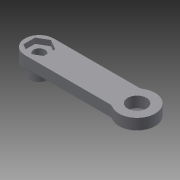
# Autodesk Inventor part: link_long
Saved by Autodesk Inventor 2014 (Build 180170000, 170)
## iProperties
Created: 2015-03-09
Part Number: link_long
Material: 一般
Document SubType Name: Modeling
Designer: Hideyuki Takei
Density: 1 g/cm^3
Appearance: 既定
Author: Hideyuki Takei
Autodesk Inventor part; units mm, degrees
note: some values were not read from the file. Chosen so that the rebuilt part matches the saved one: sketch regions of "押し出し1".
ref_plane "YZ Plane" through (0, 0, 0) normal (1, 0, 0) x (0, 1, 0)
ref_plane "XZ Plane" through (0, 0, 0) normal (0, 1, 0) x (-1, 0, 0)
ref_plane "XY Plane" through (0, 0, 0) normal (0, 0, 1) x (1, 0, 0)
sketch "スケッチ1" plane through (0, 0, 0) normal (0, 0, 1) x (1, 0, 0)
  line L0 (0, 0) -> (27.1, 0) construction
  line L1 (0, -4) -> (27.1, -4)
  line L2 (27.1, 4) -> (0, 4)
  arc A0 (0, 4) -> (0, -4) centre (0, 0) ccw
  arc A1 (27.1, -4) -> (27.1, 4) centre (27.1, 0) ccw
  circle A2 centre (0, 0) radius 1.6
  circle A3 centre (27.1, 0) radius 2.6
  circle A4 centre (27.1, 0) radius 5
  point P0 (13.55, 0)
  dimension "d0" = 27.1
  dimension "d1" = 4
  dimension "d2" = 3.2
  dimension "d3" = 5.2
  dimension "d6" = 10
  constraints: 8 end point, 5 centre point, 4 point on circle, 4 tangent, 3 coincident, 1 horizontal, 1 midpoint, 1 parallel
  measures "d0" distance of L0.start L0.end
  measures "d1" radius of A0
  measures "d2" diameter of A2
  measures "d3" diameter of A3
  measures "d6" diameter of A4
extrude "押し出し1" add sketch "スケッチ1" along normal blind 3
sketch "スケッチ3" plane through (0, 0, 0) normal (0, 0, 1) x (1, 0, 0)
  circle A0 centre (0, 0) radius 4
  circle A1 centre (0, 0) radius 1.6
  dimension "d7" = 8
  dimension "d10" = 3.2
  constraints: 2 centre point, 2 coincident
  measures "d7" diameter of A0
  measures "d10" diameter of A1
extrude "押し出し2" add sketch "スケッチ3" against normal blind 0.5
sketch "スケッチ4" plane through (0, 0, 0) normal (0, 0, 1) x (1, 0, 0)
  circle A0 centre (0, 0) radius 1.6
  circle A1 centre (0, 0) radius 2.5
  dimension "d11" = 5
  dimension "d12" = 3.2
  constraints: 2 centre point, 2 coincident
  measures "d11" diameter of A1
  measures "d12" diameter of A0
extrude "押し出し3" add sketch "スケッチ4" against normal blind 3.7
sketch "スケッチ5" plane through (0, 0, 3) normal (0, 0, 1) x (1, 0, 0)
  circle A0 centre (0, 0) radius 1.6 projected
  arc A1 (0, 4) -> (0, -4) centre (0, 0) ccw projected
  line L0 (0, 3.2332) -> (2.8, 1.6166)
  line L1 (2.8, 1.6166) -> (2.8, -1.6166)
  line L2 (2.8, -1.6166) -> (0, -3.2332)
  line L3 (0, -3.2332) -> (-2.8, -1.6166)
  line L4 (-2.8, -1.6166) -> (-2.8, 1.6166)
  line L5 (-2.8, 1.6166) -> (0, 3.2332)
  dimension "d15" = 5.6
  constraints: 12 end point, 1 coincident, 13 other
  measures "d15" distance between parallel lines of L1 L4
extrude "押し出し4" cut sketch "スケッチ5" against normal blind 1.5
fillet "フィレット1" radius 2 2 edges at (24.1, 4, 1.5) (24.1, -4, 1.5)
